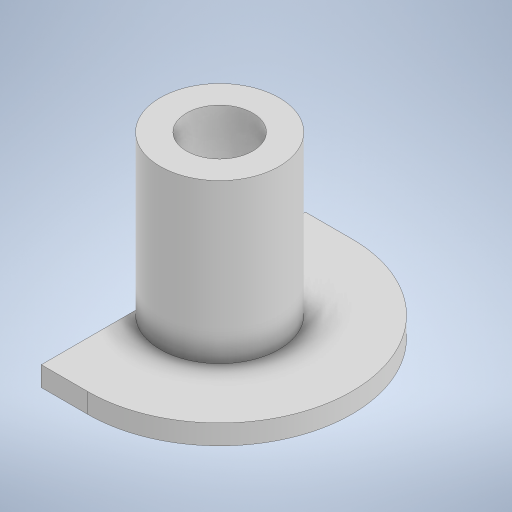
# Autodesk Inventor part: Fluorescence_fiber_holder
Saved by Autodesk Inventor 2024 (Build 280153000, 153)
## iProperties
Created: 2024-05-20
Part Number: Fluorescence_fiber_holder
Material: Generic
Document SubType Name: Modeling
Designer: david
Density: 1 g/cm^3
Appearance: Default
Author: david
Autodesk Inventor part; units mm, degrees
ref_plane "YZ Plane" through (0, 0, 0) normal (1, 0, 0) x (0, 1, 0)
ref_plane "XZ Plane" through (0, 0, 0) normal (0, 1, 0) x (-1, 0, 0)
ref_plane "XY Plane" through (0, 0, 0) normal (0, 0, 1) x (1, 0, 0)
sketch "Sketch1" plane through (0, 0, 0) normal (0, 1, 0) x (-1, 0, 0)
  circle A0 centre (0, 0) radius 10
  line L0 (0, 10) -> (0, -10)
  line L1 (0, 10) -> (3.5, 10)
  line L2 (3.5, 10) -> (3.5, -10)
  line L3 (3.5, -10) -> (0, -10)
  dimension "d0" = 20
  dimension "d3" = 3.5
  constraints: 8 end point, 2 perpendicular, 2 point on circle, 1 centre point, 1 coincident, 1 horizontal, 1 tangent, 1 vertical
  measures "d0" diameter of A0
  measures "d3" distance of L0.start L1.end
extrude "Extrusion1" add sketch "Sketch1" along normal blind 1.5 contours L0 A0 | L1 L2 A0 | A0 L2 L0 | A0 L2 L3
sketch "Sketch3" plane through (0, 1.5, 0) normal (0, 1, 0) x (1, 0, 0)
  circle A0 centre (0, 0) radius 4.5
  circle A1 centre (0, 0) radius 2.5
  dimension "d8" = 9
  dimension "d18" = 5
  constraints: 2 centre point, 2 coincident
  measures "d8" diameter of A0
  measures "d18" diameter of A1
extrude "Extrusion3" add sketch "Sketch3" along normal blind 10 and the other way blind 1.5
sketch "Sketch4" plane through (0, 11.5, 0) normal (0, 1, 0) x (1, 0, 0)
  line L0 (-3.5, 10) -> (-3.5, 2.8284) projected
  circle A0 centre (0, 0) radius 4.5
  circle A1 centre (0, 0) radius 2.5
  dimension "d13" = 5
  constraints: 2 coincident, 1 centre point, 3 other
  measures "d13" diameter of A1
extrude "Extrusion4" add sketch "Sketch4" along normal blind 2 and the other way blind 3
sketch "Sketch2" plane through (0, 1.5, 0) normal (0, 1, 0) x (1, 0, 0)
  circle A0 centre (0, 0) radius 2.5
  circle A1 centre (0, 0) radius 4.5
  dimension "d4" = 5
  dimension "d5" = 9
  constraints: 2 centre point, 2 coincident
  measures "d4" diameter of A0
  measures "d5" diameter of A1
extrude "Extrusion2" cut sketch "Sketch2" against normal blind 1.5 contours A0
body "Solid1"
